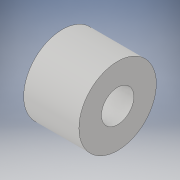
# Autodesk Inventor part: roller3 grp17
Saved by Autodesk Inventor 2019 (Build 230136000, 136)
## iProperties
Created: 2020-02-17
Part Number: roller3 grp17
Material: Generic
Document SubType Name: Modeling
Designer: Aishwarya
Density: 1 g/cm^3
Appearance: Default
Author: Aishwarya
Autodesk Inventor part; units mm, degrees
ref_plane "YZ Plane" through (0, 0, 0) normal (1, 0, 0) x (0, 1, 0)
ref_plane "XZ Plane" through (0, 0, 0) normal (0, 1, 0) x (-1, 0, 0)
ref_plane "XY Plane" through (0, 0, 0) normal (0, 0, 1) x (1, 0, 0)
sketch "Sketch1" plane through (0, 0, 0) normal (1, 0, 0) x (0, 1, 0)
  circle A0 centre (0, 0) radius 17.5
  circle A1 centre (0, 0) radius 7.3318
  dimension "d0" = 35
  constraints: 2 centre point, 2 coincident
  measures "d0" diameter of A0
extrude "Extrusion1" add sketch "Sketch1" along normal blind 25
body "Solid1"
